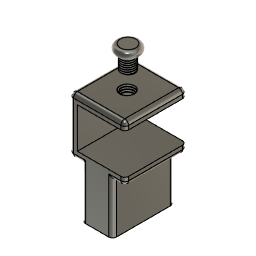
PMMA Rod Mount (Autodesk Fusion 360 design; units mm, degrees)
Autodesk Fusion 360 part; units mm, degrees
note: some values were not read from the file. Chosen so that the rebuilt part matches the saved one: which face or edge a step refers to; add or cut; where a thread starts.
imported_body "Derived Base Feature1" makes body 1 makes body 2 in component "Glass Prism Mount"
sketch "Sketch2" plane through (0, -2.75, 0) normal (0, -1, 0) x (1, 0, 0) in component "Glass Prism Mount"
  line L0 (38.1, 99.2) -> (33.1, 99.2)
  line L1 (33.1, 99.2) -> (33.1, 23)
  line L2 (33.1, 23) -> (38.1, 23)
  line L3 (38.1, 23) -> (38.1, 99.2)
  line L4 (-33.1, 99.2) -> (-38.1, 99.2) construction
  line L5 (-38.1, 99.2) -> (-38.1, 23) construction
  line L6 (-38.1, 23) -> (-33.1, 23) construction
  line L7 (-33.1, 23) -> (-33.1, 99.2) construction
  line L8 (38.1, 99.2) -> (-38.1, 99.2) construction
  line L9 (-38.1, 99.2) -> (-38.1, 23) construction
  line L10 (-38.1, 23) -> (38.1, 23) construction
  line L11 (38.1, 23) -> (38.1, 99.2) construction
  circle A0 centre (0, 61.1) radius 14
  circle A1 centre (0, 61.1) radius 19
  line L12 (0, 42.1) -> (-10, 42.1) construction
  line L13 (0, 42.1) -> (10, 42.1) construction
  line L14 (-10, 42.1) -> (-10, 44.9445)
  line L15 (10, 42.1) -> (10, 44.9445)
  line L16 (47.5, 10) -> (47.5, 96.7)
  line L17 (47.5, 96.7) -> (40.6, 96.7)
  line L18 (40.6, 96.7) -> (40.6, 20.5)
  line L19 (40.6, 20.5) -> (-40.6, 20.5)
  line L20 (-40.6, 20.5) -> (-40.6, 96.7)
  line L21 (-40.6, 96.7) -> (-47.5, 96.7)
  line L22 (-47.5, 96.7) -> (-47.5, 10)
  line L23 (-47.5, 10) -> (47.5, 10)
  line L24 (-10, 42.1) -> (-10, 10)
  line L25 (10, 42.1) -> (10, 10)
  line L26 (-10, 10) -> (10, 10)
  dimension "d3" = 28
  dimension "d4" = 38
  dimension "d5" = 10
  dimension "d6" = 10
  constraint horizontal L8
  constraint vertical L9
  constraint horizontal L10
  constraint vertical L11
  constraint coincident L5.end L6.start
  constraint coincident L0.start L3.end
  constraint concentric A0 A1
  constraint coincident A1 L12.start
  constraint perpendicular L1 L12
  constraint tangent A1 L13
  constraint parallel L12 L13
  constraint coincident A1 L14.end
  constraint perpendicular L12 L14
  constraint coincident A1 L15.end
  constraint perpendicular L13 L15
  constraint coincident L23 L24.end
  constraint perpendicular L23 L24
  constraint coincident L23 L25.end
  constraint perpendicular L23 L25
  measures "d3" diameter of A0
  measures "d4" diameter of A1
  measures "d5" distance of L12.start L12.end
  measures "d6" distance of L12.start L13.end
extrude "Extrude1" add sketch "Sketch2" along normal blind 15 separate body contours A1 | A1 L14 L15 L19 L24 L25 | L19 L23 L24 L25 L26 makes body 3 in component "Glass Prism Mount"
move_body "Move1" bodies 3 to x (1, 0, 0) y (0, 1, 0) z (0, 0, 1) at (0, -30, 0) in component "Glass Prism Mount"
ref_plane "WorkPlane1" through (0, -40.2734, 80.1) normal (0, 0, 1) x (1, 0, 0) in component "Glass Prism Mount"
sketch "Sketch3" plane through (0, -39.8774, 80.1) normal (0, 0, 1) x (1, 0, 0) in component "Glass Prism Mount"
  line L0 (-19, 7.1274) -> (19, 7.1274)
  line L1 (-19, -7.8726) -> (19, -7.8726)
  line L2 (0, 7.1274) -> (0, -7.8726) construction
  circle A0 centre (0, -0.3726) radius 5
  dimension "d10" = 10
  constraint midpoint L0 L2.start
  constraint midpoint L1 L2.end
  constraint midpoint L2 A0.centre
  measures "d10" diameter of A0
extrude "Extrude2" cut sketch "Sketch3" along normal up to surface end surface at (13.9304, -42.75, 59.7061) on bodies 3 bodies 3 in component "Glass Prism Mount"
move_body "Move2" bodies 3 to x (1, 0, 0) y (0, 1, 0) z (0, 0, 1) at (0, 0, 70) in component "Glass Prism Mount"
sketch "Sketch4" plane through (0, 0, 80) normal (0, 0, -1) x (1, 0, 0) in component "Glass Prism Mount"
  line L0 (-10, 32.75) -> (10, 32.75)
  line L1 (10, 32.75) -> (10, 47.75)
  line L2 (10, 47.75) -> (-10, 47.75)
  line L3 (-10, 47.75) -> (-10, 32.75)
  circle A0 centre (0, 40.25) radius 5.25
  dimension "d13" = 10.5
  measures "d13" diameter of A0
extrude "Extrude3" cut sketch "Sketch4" against normal blind 10 contours A0 bodies 3 in component "Glass Prism Mount"
move_body "Move3" bodies 3 to x (1, 0, 0) y (0, 1, 0) z (0, 0, 1) at (0, 0, -70) in component "Glass Prism Mount"
ref_plane "WorkPlane2" through (0, -47.5578, 80.1) normal (0, 0, 1) x (1, 0, 0) in component "Glass Prism Mount"
sketch "Sketch5" plane through (0, -46.7785, 80.1) normal (0, 0, 1) x (1, 0, 0) in component "Glass Prism Mount"
  line L0 (-19, 14.0285) -> (19, 14.0285)
  line L1 (-19, -0.9715) -> (19, -0.9715)
  line L2 (0, -0.9715) -> (0, 14.0285) construction
  circle A0 centre (0, 6.5285) radius 5
  dimension "d17" = 10
  constraint midpoint L1 L2.start
  constraint midpoint L0 L2.end
  constraint midpoint L2 A0.centre
  measures "d17" diameter of A0
sketch "Sketch6" plane through (0, -47.75, 0) normal (0, -1, 0) x (1, 0, 0) in component "Glass Prism Mount"
  circle A0 centre (0, 61.1) radius 14
  line L0 (-10, 44.9445) -> (-10, 10)
  line L1 (-10, 10) -> (10, 10)
  line L2 (10, 10) -> (10, 44.9445)
  arc A1 (10, 44.9445) -> (-10, 44.9445) centre (0, 61.1) ccw
extrude "Extrude4" add sketch "Sketch5" along normal blind 10 separate body makes body 4 in component "Glass Prism Mount"
sketch "Sketch7" plane through (0, 0, 90.1) normal (0, 0, 1) x (-1, 0, 0) in component "Glass Prism Mount"
  circle A0 centre (0, 40.25) radius 5
  circle A1 centre (0, 40.25) radius 7.5
  dimension "d20" = 15
  constraint concentric A0 A1
  measures "d20" diameter of A1
extrude "Extrude5" add sketch "Sketch7" along normal blind 5 contours A0 | A1 bodies 4 in component "Glass Prism Mount"
thread "Thread2" "ISO Metric profile 9.0 M9x1.25 6g" major diameter 8.866 minor diameter 7.4455 pitch 1.25 angle 60 modelled right hand crest width 0.1834 on face at (4.9938, -40.4992, 86.7667) crest through (4.433, -40.25, 79.7875) on bodies 4 in component "Glass Prism Mount"
move_body "Move4" bodies 3 to x (1, 0, 0) y (0, 1, 0) z (0, 0, 1) at (0, 0, 13) in component "Glass Prism Mount"
move_body "Move5" bodies 4 to x (1, 0, 0) y (0, 1, 0) z (0, 0, 1) at (0, 0, 13) in component "Glass Prism Mount"
move_body "Move6" bodies 2 to x (1, 0, 0) y (0, 1, 0) z (0, 0, 1) at (0, 0, 13) in component "Glass Prism Mount"
extrude "Extrude6" cut 1 faces at (8.4167, -40.25, 23) along direction (0, 0, -1) blind 13 on bodies 3 bodies 2 in component "Glass Prism Mount"
extrude "Extrude7" cut 2 faces at (8.4167, -40.25, 23) (8.4167, -40.25, 23) along direction (0, 0, -1) blind 13 on bodies 3 bodies 2 in component "Glass Prism Mount"
sketch "Sketch8" plane through (0, 0, 10) normal (0, 0, 1) x (-1, 0, 0) in component "Glass Prism Mount"
  line L0 (-68, 29.876) -> (-68, 34.876)
  line L1 (-68, 34.876) -> (-72, 34.876)
  line L2 (-72, 34.876) -> (-72, -34.876)
  line L3 (-72, -34.876) -> (-68, -34.876)
  line L4 (-68, -34.876) -> (-68, -29.876)
  line L5 (-68, -29.876) -> (-62, -29.876)
  line L6 (-62, -29.876) -> (-62, -50.876)
  line L7 (-62, -50.876) -> (-68, -50.876)
  line L8 (-68, -50.876) -> (-68, -45.876)
  line L9 (-68, -45.876) -> (-72, -45.876)
  line L10 (-72, -45.876) -> (-72, -72)
  line L11 (-72, -72) -> (-45.876, -72)
  line L12 (-45.876, -72) -> (-45.876, -68)
  line L13 (-45.876, -68) -> (-50.876, -68)
  line L14 (-50.876, -68) -> (-50.876, -62)
  line L15 (-50.876, -62) -> (-29.876, -62)
  line L16 (-29.876, -62) -> (-29.876, -68)
  line L17 (-29.876, -68) -> (-34.876, -68)
  line L18 (-34.876, -68) -> (-34.876, -72)
  line L19 (-34.876, -72) -> (34.876, -72)
  line L20 (34.876, -72) -> (34.876, -68)
  line L21 (34.876, -68) -> (29.876, -68)
  line L22 (29.876, -68) -> (29.876, -62)
  line L23 (29.876, -62) -> (50.876, -62)
  line L24 (50.876, -62) -> (50.876, -68)
  line L25 (50.876, -68) -> (45.876, -68)
  line L26 (45.876, -68) -> (45.876, -72)
  line L27 (45.876, -72) -> (72.5, -72)
  line L28 (72.5, -72) -> (72.5, -45.126)
  line L29 (72.5, -45.126) -> (77.75, -45.126)
  line L30 (77.75, -45.126) -> (77.75, -50.126)
  line L31 (77.75, -50.126) -> (82.25, -50.126)
  line L32 (82.25, -50.126) -> (82.25, -30.626)
  line L33 (82.25, -30.626) -> (77.75, -30.626)
  line L34 (77.75, -30.626) -> (77.75, -35.626)
  line L35 (77.75, -35.626) -> (72.5, -35.626)
  line L36 (72.5, -35.626) -> (72.5, 35.626)
  line L37 (72.5, 35.626) -> (77.75, 35.626)
  line L38 (77.75, 35.626) -> (77.75, 30.626)
  line L39 (77.75, 30.626) -> (82.25, 30.626)
  line L40 (82.25, 30.626) -> (82.25, 50.126)
  line L41 (82.25, 50.126) -> (77.75, 50.126)
  line L42 (77.75, 50.126) -> (77.75, 45.126)
  line L43 (77.75, 45.126) -> (72.5, 45.126)
  line L44 (72.5, 45.126) -> (72.5, 72.5)
  line L45 (72.5, 72.5) -> (45.126, 72.5)
  line L46 (45.126, 72.5) -> (45.126, 77.75)
  line L47 (45.126, 77.75) -> (50.126, 77.75)
  line L48 (50.126, 77.75) -> (50.126, 82.25)
  line L49 (50.126, 82.25) -> (30.626, 82.25)
  line L50 (30.626, 82.25) -> (30.626, 77.75)
  line L51 (30.626, 77.75) -> (35.626, 77.75)
  line L52 (35.626, 77.75) -> (35.626, 72.5)
  line L53 (35.626, 72.5) -> (-35.626, 72.5)
  line L54 (-35.626, 72.5) -> (-35.626, 77.75)
  line L55 (-35.626, 77.75) -> (-30.626, 77.75)
  line L56 (-30.626, 77.75) -> (-30.626, 82.25)
  line L57 (-30.626, 82.25) -> (-50.126, 82.25)
  line L58 (-50.126, 82.25) -> (-50.126, 77.75)
  line L59 (-50.126, 77.75) -> (-45.126, 77.75)
  line L60 (-45.126, 77.75) -> (-45.126, 72.5)
  line L61 (-45.126, 72.5) -> (-72, 72.5)
  line L62 (-72, 72.5) -> (-72, 45.876)
  line L63 (-72, 45.876) -> (-68, 45.876)
  line L64 (-68, 45.876) -> (-68, 50.876)
  line L65 (-68, 50.876) -> (-62, 50.876)
  line L66 (-62, 50.876) -> (-62, 29.876)
  line L67 (-62, 29.876) -> (-68, 29.876)
  circle A0 centre (40.376, 40.376) radius 5.25
  circle A1 centre (-40.376, -40.376) radius 5.25
  circle A2 centre (0, -40.376) radius 5.25
  circle A3 centre (40.376, 0) radius 5.25
  circle A4 centre (0, 40.376) radius 5.25
  circle A5 centre (-40.376, 0) radius 5.25
  circle A6 centre (40.376, -40.376) radius 5.25
  circle A7 centre (0, 0) radius 5.25
  circle A8 centre (-40.376, 40.376) radius 5.25
  line L68 (-50, 27.876) -> (50, 27.876)
  line L69 (50, 27.876) -> (50, 52.876)
  line L70 (50, 52.876) -> (-50, 52.876)
  line L71 (-50, 52.876) -> (-50, 27.876)
  line L72 (-50, 27.876) -> (50, 52.876) construction
  line L73 (50, 27.876) -> (-50, 52.876) construction
  point P0 (0, 40.376)
  dimension "d31" = 100
  dimension "d32" = 25
  constraint horizontal L68
  constraint perpendicular L68 L69
  constraint parallel L68 L70
  constraint parallel L69 L71
  constraint coincident L72 P0
  constraint coincident L73 P0
  constraint coincident P0 A4.centre
  measures "d31" distance of L69.end L70.end
  measures "d32" distance of L68.end L69.end
extrude "Extrude8" add sketch "Sketch8" along normal blind 13 separate body contours A0 | A4 | A8 | L68 L69 L70 L71 makes body 5 in component "Glass Prism Mount"
sketch "Sketch9" plane through (0, 0, 23) normal (0, 0, 1) x (-1, 0, 0) in component "Glass Prism Mount"
  line L0 (-50, 52.876) -> (-50, 27.876)
  line L1 (-50, 27.876) -> (50, 27.876)
  line L2 (50, 27.876) -> (50, 52.876)
  line L3 (50, 52.876) -> (-50, 52.876)
  circle A0 centre (-40.376, 40.376) radius 5.25
  circle A1 centre (0, 40.376) radius 5.25
  circle A2 centre (40.376, 40.376) radius 5.25
  line L4 (40.376, 35.126) -> (-40.376, 35.126)
  line L5 (-40.376, 45.626) -> (40.376, 45.626)
  constraint coincident A2 L4.start
  constraint coincident A0 L4.end
  constraint tangent A0 L4
  constraint coincident A0 L5.start
  constraint coincident A2 L5.end
  constraint tangent A2 L5
  constraint parallel L4 L5
extrude "Extrude9" cut sketch "Sketch9" against normal blind 10 contours A0 | A0 A1 L4 L5 | A1 A2 L4 L5 | A1 | A2 bodies 5 in component "Glass Prism Mount"
move_body "Move7" bodies 5 to x (1, 0, 0) y (0, 1, 0) z (0, 0, 1) at (0, 0, 10) in component "Glass Prism Mount"
move_body "Move8" bodies 3 to x (1, 0, 0) y (0, 1, 0) z (0, 0, 1) at (0, 0, 10) in component "Glass Prism Mount"
move_body "Move9" bodies 4 to x (1, 0, 0) y (0, 1, 0) z (0, 0, 1) at (0, 0, 10) in component "Glass Prism Mount"
extrude "Extrude10" add 1 faces at (16.6667, -44.5427, 20) along direction (0, 0, -1) blind 10 on bodies 5 bodies 5 in component "Glass Prism Mount"
sketch "Sketch10" plane through (0, 0, 10) normal (0, 0, -1) x (1, 0, 0) in component "Glass Prism Mount"
  line L0 (50, 27.876) -> (50, 52.876)
  line L1 (50, 52.876) -> (-50, 52.876)
  line L2 (-50, 52.876) -> (-50, 27.876)
  line L3 (-50, 27.876) -> (50, 27.876)
  circle A0 centre (40.376, 40.376) radius 5.25
  circle A1 centre (0, 40.376) radius 5.25
  circle A2 centre (-40.376, 40.376) radius 5.25
extrude "Extrude11" cut sketch "Sketch10" against normal blind 10 contours A0 | A1 | A2 bodies 5 in component "Glass Prism Mount"
extrude "Extrude12" add 1 faces at (50, -36.2093, 17.6667) along direction (1, 0, 0) blind 5 on bodies 5 bodies 5 in component "Glass Prism Mount"
extrude "Extrude13" add 1 faces at (-50, -36.2093, 25.3333) along direction (-1, 0, 0) blind 5 on bodies 5 bodies 5 in component "Glass Prism Mount"
fillet "Fillet3" radius 12.5 4 edges at (55, -52.876, 21.5) (55, -27.876, 21.5) (-55, -52.876, 21.5) (-55, -27.876, 21.5) on bodies 5 in component "Glass Prism Mount"
extrude "Extrude14" cut 1 faces at (0.3487, -32.75, 45.3797) along direction (0, 1, 0) blind 0.375 on bodies 3 bodies 2 in component "Glass Prism Mount"
extrude "Extrude15" cut 1 faces at (0.3487, -32.75, 45.3797) along direction (0, -1, 0) blind 0.375 on bodies 3 bodies 2 in component "Glass Prism Mount"
extrude "Extrude16" cut 1 faces at (0.3487, -32.75, 45.3797) along direction (0, 1, 0) blind 0.375 on bodies 3 bodies 2 in component "Glass Prism Mount"
extrude "Extrude17" cut 1 faces at (0.3487, -32.75, 45.3797) along direction (0, -1, 0) blind 0.375 on bodies 3 bodies 2 in component "Glass Prism Mount"
extrude "Extrude18" cut 1 faces at (0.3487, -32.75, 45.3797) along direction (0, -1, 0) blind 0.125 on bodies 3 bodies 2 in component "Glass Prism Mount"
extrude "Extrude19" cut 1 faces at (0.3487, -32.75, 45.3797) along direction (0, 1, 0) blind 0.125 on bodies 3 bodies 2 in component "Glass Prism Mount"
extrude "Extrude20" cut 1 faces at (0.3487, -32.75, 45.3797) along direction (0, 1, 0) blind 0.125 on bodies 3 bodies 2 in component "Glass Prism Mount"
extrude "Extrude21" cut 1 faces at (0.3487, -32.75, 45.3797) along direction (0, -1, 0) blind 0.125 on bodies 3 bodies 2 in component "Glass Prism Mount"
sketch "Sketch1" plane through (0, -47.75, 0) normal (0, -1, 0) x (1, 0, 0)
  circle A0 centre (0, 84.1) radius 14
  line L0 (-10, 67.9445) -> (-10, 33)
  line L1 (-10, 33) -> (10, 33)
  line L2 (10, 33) -> (10, 67.9445)
  arc A1 (10, 67.9445) -> (-10, 67.9445) centre (0, 84.1) ccw
  line L3 (12.875, 97.175) -> (-12.875, 97.175)
  line L4 (-12.875, 97.175) -> (-12.875, 71.025)
  line L5 (-12.875, 71.025) -> (12.875, 71.025)
  line L6 (12.875, 71.025) -> (12.875, 97.175)
  line L7 (12.875, 97.175) -> (-12.875, 71.025) construction
  line L8 (-12.875, 97.175) -> (12.875, 71.025) construction
  line L9 (-17.875, 102.175) -> (17.875, 102.175)
  line L10 (17.875, 102.175) -> (17.875, 66.025)
  line L11 (17.875, 66.025) -> (-17.875, 66.025)
  line L12 (-17.875, 66.025) -> (-17.875, 102.175)
  line L13 (-17.875, 102.175) -> (17.875, 66.025) construction
  line L14 (17.875, 102.175) -> (-17.875, 66.025) construction
  point P0 (0, 84.1)
  point P1 (0, 84.1)
  dimension "d63" = 25.75
  dimension "d64" = 26.15
  dimension "d65" = 35.75
  dimension "d66" = 36.15
  constraint horizontal L3
  constraint perpendicular L3 L4
  constraint parallel L3 L5
  constraint parallel L4 L6
  constraint coincident L7 P1
  constraint coincident L8 P1
  constraint coincident P0 A0.centre
  constraint horizontal L9
  constraint perpendicular L9 L10
  constraint parallel L9 L11
  constraint parallel L10 L12
  constraint coincident L13 P1
  constraint coincident L14 P1
  constraint coincident P1 P0
  measures "d63" distance of L4.end L5.end
  measures "d64" distance of L3.end L4.end
  measures "d65" distance of L10.end L11.end
  measures "d66" distance of L9.end L10.end
extrude "Extrude22" cut sketch "Sketch1" against normal blind 15 contours A0 L3 L6 | A0 L5 L6 | A0 L3 L4 | A0 L4 L5 bodies 3 in component "Glass Prism Mount"
extrude "Extrude23" add sketch "Sketch1" against normal blind 15 contours A0 L6 | A0 L3 | A0 L5 | A0 L4 | L0 A1 L11 L12 | L2 A1 L10 L11 | A1 L9 L12 | A1 L9 L10 bodies 3 in component "Glass Prism Mount"
move_body "Move10" bodies 4 to x (1, 0, 0) y (0, 1, 0) z (0, 0, 1) at (0, 0, 10) in component "Glass Prism Mount"
extrude "Extrude24" cut sketch "Sketch1" against normal blind 15 contours A1 L12 | A1 L9 | A1 L10 bodies 3 in component "Glass Prism Mount"
sketch "Sketch2 (2)" plane through (0, 0, 97.175) normal (0, 0, -1) x (1, 0, 0)
  line L0 (12.875, 47.75) -> (-12.875, 47.75)
  line L1 (-12.875, 47.75) -> (-12.875, 32.75)
  line L2 (-12.875, 32.75) -> (12.875, 32.75)
  line L3 (12.875, 32.75) -> (12.875, 47.75)
  line L4 (0, 32.75) -> (0, 40.25) construction
  circle A0 centre (0, 40.25) radius 5
  dimension "d73" = 7.5
  dimension "d74" = 10
  constraint midpoint L2 L4.start
  constraint perpendicular L0 L4
  constraint coincident L4.end A0.centre
  measures "d73" distance of L4.start L4.end
  measures "d74" diameter of A0
extrude "Extrude25" cut sketch "Sketch2 (2)" against normal blind 5 contours A0 bodies 3 in component "Glass Prism Mount"
thread "Thread3" "ISO Metric profile 10.0 M10x1.5 6H" major diameter 10.198 minor diameter 8.526 pitch 1.5 angle 60 modelled right hand crest width 0.4094 on face at (-4.9848, -39.8601, 100.5112) crest through (4.263, -40.25, 103.3) on bodies 3 in component "Glass Prism Mount"
extrude "Extrude26" add 1 faces at (-3.3333, -32.75, 44.0083) along direction (0, 1, 0) blind 12.5 on bodies 3 bodies 3 in component "Glass Prism Mount"
extrude "Extrude27" add 1 faces at (-3.3333, -47.75, 44.0083) along direction (0, -1, 0) blind 12.5 on bodies 3 bodies 3 in component "Glass Prism Mount"
fillet "Fillet4" radius 2.5 14 edges at (17.875, -60.25, 84.1) (0, -60.25, 102.175) (-17.875, -60.25, 84.1) (-13.9375, -60.25, 66.025) (13.9375, -60.25, 66.025) (10, -60.25, 49.5125) (-10, -60.25, 49.5125) (17.875, -20.25, 84.1) (0, -20.25, 102.175) (-17.875, -20.25, 84.1) (-13.9375, -20.25, 66.025) (13.9375, -20.25, 66.025) (10, -20.25, 49.5125) (-10, -20.25, 49.5125) on bodies 3 4 in component "Glass Prism Mount"
fillet "Fillet4" radius 2.5 4 edges at (-17.875, -40.25, 102.175) (-17.875, -40.25, 66.025) (17.875, -40.25, 102.175) (17.875, -40.25, 66.025) on bodies 3 4 in component "Glass Prism Mount"
fillet "Fillet4" radius 2.5 2 edges at (6.9925, -37.5379, 128.1) (6.9925, -37.5379, 123.1) on bodies 3 4 in component "Glass Prism Mount"
extrude "Extrude28" cut 1 faces at (12.875, -46.9167, 79.7417) along direction (1, 0, 0) blind 5 on bodies 3 bodies 3 in component "Glass Prism Mount"
component "Glass Prism Mount" placed x (1, 0, 0) y (0, 1, 0) z (0, 0, 1) at (0, 0, 0)
hidden bodies 1 2 5
equation "d65 = 25.750 mm + 10 mm"
equation "d66 = 26.150 mm + 10 mm"
named bodies: "Optical Breadboard", "Mirror Slot Post"
